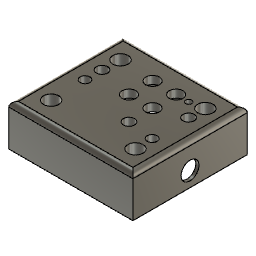
project (Autodesk Fusion 360 archive; units mm, degrees)
design "Obudowa"
Autodesk Fusion 360 part; units mm, degrees
sketch "Sketch1" plane through (0, 0, 0) normal (0, 0, 1) x (1, 0, 0)
  line L0 (-25, 25) -> (28.34, 25)
  line L1 (28.34, 25) -> (28.34, -20.72)
  line L2 (28.34, -20.72) -> (-25, -20.72)
  line L3 (-25, -20.72) -> (-25, 25)
  circle A0 centre (-19.67, -15.64) radius 1.6
  circle A1 centre (23.26, -15.64) radius 1.6
  circle A2 centre (23.26, 19.92) radius 1.6
  circle A3 centre (-19.793, 19.793) radius 1.6
  dimension "d1" = 53.34
  dimension "d2" = 45.72
  dimension "d3" = 3.2
  dimension "d4" = 5.08
  dimension "d5" = 5.33
  dimension "d6" = 3.2
  dimension "d7" = 3.2
  dimension "d8" = 3.2
  dimension "d9" = 5.08
  dimension "d10" = 5.08
  dimension "d11" = 5.207
  dimension "d12" = 5.207
  dimension "d13" = 5.08
  dimension "d14" = 5.08
  constraint horizontal L0
  constraint vertical L1
  constraint horizontal L2
  constraint vertical L3
  measures "d1" distance of L0.start L0.end
  measures "d2" distance of L0.start L2.end
  measures "d3" diameter of A0
  measures "d4" distance of L2 A0.centre
  measures "d5" distance of L3 A0.centre
  measures "d6" diameter of A1
  measures "d7" diameter of A2
  measures "d8" diameter of A3
  measures "d9" distance of L2 A1.centre
  measures "d10" distance of L0 A2.centre
  measures "d11" distance of L0 A3.centre
  measures "d12" distance of L3 A3.centre
  measures "d13" distance of L1 A2.centre
  measures "d14" distance of L1 A1.centre
extrude "Extrude1" add sketch "Sketch1" along normal blind 1.6 makes body 1
sketch "Sketch2" plane through (0, 0, 1.6) normal (0, 0, 1) x (-1, 0, 0)
  circle A0 centre (19.793, -19.793) radius 1.6
  circle A1 centre (-23.26, -19.92) radius 1.6
  circle A2 centre (-23.26, 15.64) radius 1.6
  circle A3 centre (19.67, 15.64) radius 1.6
  line L0 (25, 20.72) -> (-28.34, 20.72)
  line L1 (-28.34, 20.72) -> (-28.34, -25)
  line L2 (-28.34, -25) -> (25, -25)
  line L3 (25, -25) -> (25, 20.72)
  circle A4 centre (-3.94, -17.13) radius 2.2
  circle A5 centre (-11.8, 15.89) radius 4.25
  circle A6 centre (7.98, 9.3) radius 2.25
  dimension "d17" = 4.4
  dimension "d18" = 7.87
  dimension "d19" = 28.94
  dimension "d20" = 8.5
  dimension "d21" = 4.83
  dimension "d22" = 16.54
  dimension "d23" = 4.5
  dimension "d24" = 17.02
  dimension "d25" = 11.42
  measures "d17" diameter of A4
  measures "d18" distance of L2 A4.centre
  measures "d19" distance of L3 A4.centre
  measures "d20" diameter of A5
  measures "d21" distance of L0 A5.centre
  measures "d22" distance of L1 A5.centre
  measures "d23" diameter of A6
  measures "d24" distance of L3 A6.centre
  measures "d25" distance of L0 A6.centre
extrude "Extrude2" add sketch "Sketch2" along normal blind 12 contours A5 bodies 1
extrude "Extrude3" add sketch "Sketch2" along normal blind 8 contours A4 bodies 1
extrude "Extrude4" add sketch "Sketch2" along normal blind 8 contours A6 bodies 1
sketch "Sketch3" plane through (0, 0, 1.6) normal (0, 0, 1) x (-1, 0, 0)
  circle A0 centre (-18.865, -2.105) radius 1.65
  line L0 (-28.34, -25) -> (25, -25)
  line L1 (-28.34, 20.72) -> (-28.34, -25)
  circle A1 centre (-18.865, -2.105) radius 3.555
  line L2 (-18.865, -2.105) -> (-27.075, -2.105)
  line L3 (-27.075, -2.105) -> (-27.075, 1.45)
  line L4 (-27.075, 1.45) -> (-18.865, 1.45)
  line L5 (-18.865, 1.45) -> (-18.865, -2.105)
  line L6 (-18.865, -2.105) -> (-27.075, -2.105)
  line L7 (-27.075, -2.105) -> (-27.075, -5.66)
  line L8 (-27.075, -5.66) -> (-18.865, -5.66)
  line L9 (-18.865, -5.66) -> (-18.865, -2.105)
  dimension "d32" = 3.3
  dimension "d33" = 22.895
  dimension "d34" = 9.475
  dimension "d35" = 7.11
  dimension "d36" = 8.21
  dimension "d37" = 3.555
  dimension "d38" = 8.21
  dimension "d39" = 3.555
  constraint concentric A0 A1
  constraint horizontal L2
  constraint vertical L3
  constraint horizontal L4
  constraint vertical L5
  constraint coincident A0.centre A1.centre
  constraint horizontal L6
  constraint vertical L7
  constraint horizontal L8
  constraint vertical L9
  measures "d32" diameter of A0
  measures "d33" distance of A0.centre L0
  measures "d34" distance of A0.centre L1
  measures "d35" diameter of A1
  measures "d36" distance of A0.centre L2.end
  measures "d37" distance of A0.centre L4.end
  measures "d38" distance of A0.centre L2.end
  measures "d39" distance of A0.centre L8.end
extrude "Extrude5" add sketch "Sketch3" along normal blind 4.7 contours A0 A1 L5 L9 | A0 A1 L2 L5 L6 | A0 A1 L2 L6 L9 | A1 L2 L3 L4 L6 | A1 L2 L6 L7 L8 bodies 1
sketch "Sketch4" plane through (0, 0, 6.3) normal (0, 0, 1) x (-1, 0, 0)
  circle A0 centre (-18.865, -2.105) radius 1.65
  line L0 (-27.075, 1.45) -> (-27.075, -5.66)
  line L1 (-27.075, -5.66) -> (-18.865, -5.66)
  arc A1 (-18.865, -5.66) -> (-18.865, 1.45) centre (-18.865, -2.105) ccw
  line L2 (-18.865, 1.45) -> (-27.075, 1.45)
  line L3 (-25.3616, 1.45) -> (-28.1165, 1.45)
  line L4 (-28.1165, 1.45) -> (-28.1165, -5.66)
  line L5 (-28.1165, -5.66) -> (-25.3616, -5.66)
  line L6 (-25.3616, -5.66) -> (-25.3616, 1.45)
  dimension "d42" = 7.11
  constraint horizontal L3
  constraint vertical L4
  constraint horizontal L5
  constraint vertical L6
  constraint coincident L2 L3.start
  measures "d42" distance of L3.start L5.end
extrude "Extrude6" add sketch "Sketch4" along normal blind 5.71 contours L0 L1 L2 L3 L5 L6 | L0 L3 L4 L5 bodies 1
sketch "Sketch5" plane through (28.1165, 0, 0) normal (1, 0, 0) x (0, 1, 0)
  line L0 (-1.45, 6.3) -> (5.66, 6.3)
  line L1 (5.66, 6.3) -> (5.66, 12.01)
  line L2 (5.66, 12.01) -> (-1.45, 12.01)
  line L3 (-1.45, 12.01) -> (-1.45, 6.3)
  circle A0 centre (2.105, 8.58) radius 4.57
  line L4 (-20.72, 1.6) -> (25, 1.6)
  dimension "d45" = 9.14
  dimension "d46" = 3.555
  dimension "d47" = 6.98
  measures "d45" diameter of A0
  measures "d46" distance of L1 A0.centre
  measures "d47" distance of A0.centre L4
extrude "Extrude7" add sketch "Sketch5" along normal blind 15 contours L0 L1 L2 L3 A0 | L0 L1 L3 A0 | L2 A0 bodies 1
extrude "Extrude8" cut 1 faces at (26.2799, 3.1116, 12.01) along direction (0, 0, -1) blind 1.5 on bodies 1 bodies 1
sketch "FRONT" plane through (0, 0, 0) normal (0, 0, 1) x (1, 0, 0)
  line L0 (-28.33, 29.64) -> (31.67, 29.64)
  line L1 (31.67, 29.64) -> (31.67, -25.36)
  line L2 (31.67, -25.36) -> (-28.33, -25.36)
  line L3 (-28.33, -25.36) -> (-28.33, 29.64)
  line L4 (28.34, 25) -> (-25, 25)
  line L5 (28.34, -20.72) -> (28.34, 25)
  circle A0 centre (-2.33, 18.64) radius 3.45
  circle A1 centre (9.67, 18.64) radius 3.45
  circle A2 centre (-2.33, 6.64) radius 3.45
  circle A3 centre (9.67, 6.64) radius 3.45
  circle A4 centre (9.67, -5.36) radius 2.85
  circle A5 centre (22.9915, 11.64) radius 2.85
  circle A6 centre (16.0978, 18.6108) radius 1.55
  circle A7 centre (22.9591, -6.8283) radius 2.5
  circle A8 centre (-20.0454, 10.64) radius 2.85
  circle A9 centre (-20.0454, 1.9723) radius 2.5
  line L6 (-16, 15) -> (-16, 13) construction
  line L7 (-16, 13) -> (-14, 13) construction
  line L8 (-14, 13) -> (-14, 15) construction
  line L9 (-14, 15) -> (-16, 15) construction
  line L10 (26, -8) -> (26, -10) construction
  line L11 (26, -10) -> (27, -10) construction
  line L12 (27, -10) -> (27, -8) construction
  line L13 (27, -8) -> (26, -8) construction
  line L14 (26, 15) -> (26, 14) construction
  line L15 (26, 14) -> (27, 14) construction
  line L16 (27, 14) -> (27, 15) construction
  line L17 (27, 15) -> (26, 15) construction
  line L18 (9, 2) -> (9, 0) construction
  line L19 (9, 0) -> (10, 0) construction
  line L20 (10, 0) -> (10, 2) construction
  line L21 (10, 2) -> (9, 2) construction
  circle A10 centre (-19.67, -15.64) radius 1.6
  circle A11 centre (23.26, -15.64) radius 1.6
  circle A12 centre (23.26, 19.92) radius 1.6
  circle A13 centre (-19.79, 19.79) radius 1.6
  circle A14 centre (-19.79, 19.79) radius 3.85
  circle A15 centre (-19.79, 19.79) radius 5
  circle A16 centre (23.26, 19.92) radius 3.85
  circle A17 centre (23.26, 19.92) radius 5
  circle A18 centre (23.26, -15.64) radius 3.85
  circle A19 centre (23.26, -15.64) radius 5
  circle A20 centre (-19.67, -15.64) radius 3.85
  circle A21 centre (-19.67, -15.64) radius 5
  line L22 (-28.33, -25.36) -> (-29.93, -25.36)
  line L23 (-29.93, -25.36) -> (-29.93, 29.64)
  line L24 (-29.93, 29.64) -> (-28.33, 29.64)
  line L25 (-28.33, 29.64) -> (-28.33, -25.36)
  line L26 (-29.93, 29.64) -> (31.67, 29.64)
  line L27 (31.67, 29.64) -> (31.67, 31.24)
  line L28 (31.67, 31.24) -> (-29.93, 31.24)
  line L29 (-29.93, 31.24) -> (-29.93, 29.64)
  line L30 (31.67, 31.24) -> (33.27, 31.24)
  line L31 (33.27, 31.24) -> (33.27, -25.36)
  line L32 (33.27, -25.36) -> (31.67, -25.36)
  line L33 (31.67, -25.36) -> (31.67, 31.24)
  line L34 (-29.93, -25.36) -> (33.27, -25.36)
  line L35 (33.27, -25.36) -> (33.27, -26.96)
  line L36 (33.27, -26.96) -> (-29.93, -26.96)
  line L37 (-29.93, -26.96) -> (-29.93, -25.36)
  dimension "d52" = 60
  dimension "d53" = 55
  dimension "d54" = 4.64
  dimension "d55" = 3.33
  dimension "d56" = 6.9
  dimension "d59" = 6.9
  dimension "d60" = 12
  dimension "d62" = 6.9
  dimension "d63" = 6.9
  dimension "d64" = 12
  dimension "d65" = 5.7
  dimension "d66" = 12
  dimension "d67" = 5.7
  dimension "d68" = 3.1
  dimension "d69" = 5
  dimension "d70" = 5.7
  dimension "d71" = 5
  dimension "d72" = 3.2
  dimension "d73" = 3.2
  dimension "d74" = 3.2
  dimension "d75" = 3.2
  dimension "d76" = 7.7
  dimension "d77" = 10
  dimension "d78" = 7.7
  dimension "d79" = 10
  dimension "d80" = 7.7
  dimension "d81" = 10
  dimension "d82" = 7.7
  dimension "d83" = 10
  dimension "d92" = 1.6
  dimension "d93" = 55
  dimension "d94" = 61.6
  dimension "d95" = 1.6
  dimension "d96" = 1.6
  dimension "d97" = 56.6
  dimension "d98" = 63.2
  dimension "d99" = 1.6
  constraint horizontal L0
  constraint vertical L1
  constraint horizontal L2
  constraint vertical L3
  constraint concentric A13 A14
  constraint concentric A13 A15
  constraint concentric A12 A16
  constraint concentric A12 A17
  constraint concentric A11 A18
  constraint concentric A18 A19
  constraint concentric A10 A20
  constraint concentric A10 A21
  constraint horizontal L22
  constraint vertical L23
  constraint horizontal L24
  constraint vertical L25
  constraint horizontal L26
  constraint vertical L27
  constraint horizontal L28
  constraint vertical L29
  constraint horizontal L30
  constraint vertical L31
  constraint horizontal L32
  constraint vertical L33
  constraint horizontal L34
  constraint vertical L35
  constraint horizontal L36
  constraint vertical L37
  measures "d52" distance of L0.start L0.end
  measures "d53" distance of L0.start L2.end
  measures "d54" distance of L0 L4
  measures "d55" distance of L1 L5
  measures "d56" diameter of A0
  measures "d59" diameter of A1
  measures "d60" horizontal distance of A0.centre A1.centre
  measures "d62" diameter of A2
  measures "d63" diameter of A3
  measures "d64" horizontal distance of A3.centre A2.centre
  measures "d65" diameter of A4
  measures "d66" distance of A3.centre A4.centre
  measures "d67" diameter of A5
  measures "d68" diameter of A6
  measures "d69" diameter of A7
  measures "d70" diameter of A8
  measures "d71" diameter of A9
  measures "d72" diameter of A10
  measures "d73" diameter of A11
  measures "d74" diameter of A12
  measures "d75" diameter of A13
  measures "d76" diameter of A14
  measures "d77" diameter of A15
  measures "d78" diameter of A16
  measures "d79" diameter of A17
  measures "d80" diameter of A18
  measures "d81" diameter of A19
  measures "d82" diameter of A20
  measures "d83" diameter of A21
  measures "d92" distance of L2.end L22.end
  measures "d93" distance of L2.end L0.start
  measures "d94" distance of L23.end L0.end
  measures "d95" distance of L23.end L28.end
  measures "d96" distance of L27.end L30.end
  measures "d97" distance of L27.end L1.end
  measures "d98" distance of L22.end L31.end
  measures "d99" distance of L22.end L36.end
move_body "Move1" bodies 1 to x (1, 0, 0) y (0, 1, 0) z (0, 0, 1) at (0, 0, -18)
extrude "Extrude9" add sketch "FRONT" along normal blind 4 separate body contours L0 L1 L2 L3 L25 L26 L33 L34 | A15 | A17 | A19 | A21 makes body 2
move_body "Move2" bodies 1 to x (1, 0, 0) y (0, 1, 0) z (0, 0, 1) at (0, 0, -20)
extrude "Extrude10" add sketch "FRONT" against normal blind 16.4 contours A10 | A11 | A12 | A13 | A14 | A15 | A16 | A17 | A18 | A19 | A20 | A21 bodies 2
extrude "Extrude11" cut sketch "FRONT" against normal blind 34 contours A10 | A11 | A12 | A13 bodies 2
extrude "Extrude12" cut sketch "FRONT" against normal blind 15.8 contours A14 | A16 | A18 | A20 bodies 2
move_body "Move3" bodies 1 to x (1, 0, 0) y (0, 1, 0) z (0, 0, 1) at (0, 0, 20)
extrude "Extrude13" add sketch "FRONT" along normal blind 4 contours L0 L24 L26 L27 L28 L29 L33 | L3 L22 L23 L24 L25 L26 L34 | L1 L27 L30 L31 L32 L33 L34 | L2 L22 L32 L34 L35 L36 L37 bodies 2
extrude "Extrude14" add sketch "FRONT" against normal blind 17 separate body contours L0 L24 L26 L27 L28 L29 L33 | L3 L22 L23 L24 L25 L26 L34 | L1 L27 L30 L31 L32 L33 L34 | L2 L22 L32 L34 L35 L36 L37 makes body 3
combine "Combine1" operation add target body 3 tool bodies 2
sketch "Sketch7" plane through (0, 0, 0) normal (0, 0, -1) x (1, 0, 0)
  circle A0 centre (-2.33, -18.64) radius 3.45
  circle A1 centre (9.67, -18.64) radius 3.45
  circle A2 centre (-2.33, -6.64) radius 3.45
  circle A3 centre (9.67, -6.64) radius 3.45
  circle A4 centre (9.67, 5.36) radius 2.85
  circle A5 centre (22.9915, -11.64) radius 2.85
  circle A6 centre (16.0978, -18.6108) radius 1.55
  circle A7 centre (22.9591, 6.8283) radius 2.5
  circle A8 centre (-20.0454, -10.64) radius 2.85
  circle A9 centre (-20.0454, -1.9723) radius 2.5
  circle A10 centre (-19.79, -19.79) radius 5
  circle A11 centre (23.26, -19.92) radius 5
  circle A12 centre (-19.67, 15.64) radius 5
  circle A13 centre (23.26, 15.64) radius 5
  line L0 (-28.33, -29.64) -> (31.67, -29.64)
  line L1 (31.67, -29.64) -> (31.67, 25.36)
  line L2 (31.67, 25.36) -> (-28.33, 25.36)
  line L3 (-28.33, 25.36) -> (-28.33, -29.64)
  line L4 (23.26, -19.92) -> (22.46, -19.92)
  line L5 (22.46, -19.92) -> (22.46, -29.991)
  line L6 (22.46, -29.991) -> (23.26, -29.991)
  line L7 (23.26, -29.991) -> (23.26, -19.92)
  line L8 (23.26, -19.92) -> (24.06, -19.92)
  line L9 (24.06, -19.92) -> (24.06, -29.991)
  line L10 (24.06, -29.991) -> (23.26, -29.991)
  line L11 (23.26, -29.991) -> (23.26, -19.92)
  line L12 (23.26, -19.92) -> (32.3548, -19.92)
  line L13 (32.3548, -19.92) -> (32.3548, -20.72)
  line L14 (32.3548, -20.72) -> (23.26, -20.72)
  line L15 (23.26, -20.72) -> (23.26, -19.92)
  line L16 (23.26, -19.92) -> (32.3548, -19.92)
  line L17 (32.3548, -19.92) -> (32.3548, -19.12)
  line L18 (32.3548, -19.12) -> (23.26, -19.12)
  line L19 (23.26, -19.12) -> (23.26, -19.92)
  line L20 (32.3548, -19.92) -> (32.3548, -19.12)
  line L21 (23.26, 15.64) -> (22.46, 15.64)
  line L22 (22.46, 15.64) -> (22.46, 26.0742)
  line L23 (22.46, 26.0742) -> (23.26, 26.0742)
  line L24 (23.26, 26.0742) -> (23.26, 15.64)
  line L25 (24.06, 26.0742) -> (24.06, 15.64)
  line L26 (24.06, 15.64) -> (23.26, 15.64)
  line L27 (23.26, 15.64) -> (23.26, 26.0742)
  line L28 (23.26, 26.0742) -> (24.06, 26.0742)
  line L29 (23.26, 15.64) -> (32.1877, 15.64)
  line L30 (32.1877, 15.64) -> (32.1877, 14.84)
  line L31 (32.1877, 14.84) -> (23.26, 14.84)
  line L32 (23.26, 14.84) -> (23.26, 15.64)
  line L33 (23.26, 15.64) -> (32.1877, 15.64)
  line L34 (32.1877, 15.64) -> (32.1877, 16.44)
  line L35 (32.1877, 16.44) -> (23.26, 16.44)
  line L36 (23.26, 16.44) -> (23.26, 15.64)
  line L37 (-19.67, 15.64) -> (-30.1363, 15.64)
  line L38 (-30.1363, 15.64) -> (-30.1363, 14.84)
  line L39 (-30.1363, 14.84) -> (-19.67, 14.84)
  line L40 (-19.67, 14.84) -> (-19.67, 15.64)
  line L41 (-19.67, 15.64) -> (-30.1363, 15.64)
  line L42 (-30.1363, 15.64) -> (-30.1363, 16.44)
  line L43 (-30.1363, 16.44) -> (-19.67, 16.44)
  line L44 (-19.67, 16.44) -> (-19.67, 15.64)
  line L45 (-19.67, 15.64) -> (-18.87, 15.64)
  line L46 (-18.87, 15.64) -> (-18.87, 25.7874)
  line L47 (-18.87, 25.7874) -> (-19.67, 25.7874)
  line L48 (-19.67, 25.7874) -> (-19.67, 15.64)
  line L49 (-19.67, 15.64) -> (-20.47, 15.64)
  line L50 (-20.47, 15.64) -> (-20.47, 25.7874)
  line L51 (-20.47, 25.7874) -> (-19.67, 25.7874)
  line L52 (-19.67, 25.7874) -> (-19.67, 15.64)
  line L53 (-19.79, -19.79) -> (-20.59, -19.79)
  line L54 (-20.59, -19.79) -> (-20.59, -30.5224)
  line L55 (-20.59, -30.5224) -> (-19.79, -30.5224)
  line L56 (-19.79, -30.5224) -> (-19.79, -19.79)
  line L57 (-19.79, -19.79) -> (-18.99, -19.79)
  line L58 (-18.99, -19.79) -> (-18.99, -30.5512)
  line L59 (-18.99, -30.5512) -> (-19.79, -30.5512)
  line L60 (-19.79, -30.5512) -> (-19.79, -19.79)
  line L61 (-19.79, -19.79) -> (-29.2063, -19.79)
  line L62 (-29.2063, -19.79) -> (-29.2063, -20.59)
  line L63 (-29.2063, -20.59) -> (-19.79, -20.59)
  line L64 (-19.79, -20.59) -> (-19.79, -19.79)
  line L65 (-19.79, -19.79) -> (-29.2063, -19.79)
  line L66 (-29.2063, -19.79) -> (-29.2063, -18.99)
  line L67 (-29.2063, -18.99) -> (-19.79, -18.99)
  line L68 (-19.79, -18.99) -> (-19.79, -19.79)
  dimension "d104" = 0.8
  dimension "d105" = 0.8
  dimension "d106" = 0.8
  dimension "d107" = 0.8
  dimension "d108" = 0.8
  dimension "d109" = 0.8
  dimension "d110" = 0.8
  dimension "d111" = 0.8
  dimension "d112" = 0.8
  dimension "d113" = 0.8
  dimension "d114" = 0.8
  dimension "d115" = 0.8
  dimension "d116" = 0.8
  dimension "d117" = 0.8
  dimension "d118" = 0.8
  constraint horizontal L4
  constraint vertical L5
  constraint horizontal L6
  constraint vertical L7
  constraint coincident A11.centre L4.start
  constraint horizontal L8
  constraint vertical L9
  constraint horizontal L10
  constraint vertical L11
  constraint horizontal L12
  constraint vertical L13
  constraint horizontal L14
  constraint vertical L15
  constraint horizontal L16
  constraint vertical L17
  constraint horizontal L18
  constraint vertical L19
  constraint vertical L20
  constraint horizontal L21
  constraint vertical L22
  constraint horizontal L23
  constraint vertical L24
  constraint coincident A13.centre L21.start
  constraint horizontal L26
  constraint vertical L27
  constraint horizontal L28
  constraint vertical L25
  constraint horizontal L29
  constraint vertical L30
  constraint horizontal L31
  constraint vertical L32
  constraint horizontal L33
  constraint vertical L34
  constraint horizontal L35
  constraint vertical L36
  constraint horizontal L37
  constraint vertical L38
  constraint horizontal L39
  constraint vertical L40
  constraint coincident A12.centre L37.start
  constraint horizontal L41
  constraint vertical L42
  constraint horizontal L43
  constraint vertical L44
  constraint horizontal L45
  constraint vertical L46
  constraint horizontal L47
  constraint vertical L48
  constraint horizontal L49
  constraint vertical L50
  constraint horizontal L51
  constraint vertical L52
  constraint horizontal L53
  constraint vertical L54
  constraint horizontal L55
  constraint vertical L56
  constraint coincident A10.centre L53.start
  constraint horizontal L57
  constraint vertical L58
  constraint horizontal L59
  constraint vertical L60
  constraint horizontal L61
  constraint vertical L62
  constraint horizontal L63
  constraint vertical L64
  constraint horizontal L65
  constraint vertical L66
  constraint horizontal L67
  constraint vertical L68
  measures "d104" distance of A11.centre L4.end
  measures "d105" distance of A11.centre L8.end
  measures "d106" distance of A11.centre L14.end
  measures "d107" distance of A11.centre L18.end
  measures "d108" distance of A13.centre L21.end
  measures "d109" distance of A13.centre L25.end
  measures "d110" distance of A13.centre L31.end
  measures "d111" distance of A13.centre L35.end
  measures "d112" distance of A12.centre L39.end
  measures "d113" distance of A12.centre L43.end
  measures "d114" distance of A12.centre L45.end
  measures "d115" distance of A12.centre L49.end
  measures "d116" distance of A10.centre L53.end
  measures "d117" distance of A10.centre L63.end
  measures "d118" distance of A10.centre L67.end
extrude "Extrude15" add sketch "Sketch7" along normal blind 15 contours A10 L3 L61 L65 L67 | A10 L0 L56 L58 L60 | A10 L3 L61 L63 L65 | A10 L0 L54 L56 L60 | A12 L3 L37 L39 L41 | A11 L0 L5 L7 L11 | A12 L3 L37 L41 L43 | A11 L0 L7 L9 L11 | A11 L1 L12 L16 L18 | A12 L2 L46 L48 L52 | A11 L1 L12 L14 L16 | A12 L2 L48 L50 L52 | A13 L1 L29 L31 L33 | A13 L2 L22 L24 L27 | A13 L1 L29 L33 L35 | A13 L2 L24 L25 L27 bodies 3
fillet "Fillet1" radius 2.5 4 edges at (1.67, -26.96, 4) (-29.93, 2.14, 4) (1.67, 31.24, 4) (33.27, 2.14, 4) on bodies 3
move_body "Move4" bodies 1 3 to x (1, 0, 0) y (0, 1, 0) z (0, 0, 1) at (0, 0, 18)
sketch "Sketch8" plane through (0, 0, 0) normal (0, 0, 1) x (1, 0, 0)
  line L0 (-29.93, -26.96) -> (33.27, -26.96)
  line L1 (33.27, -26.96) -> (33.27, 31.24)
  line L2 (33.27, 31.24) -> (-29.93, 31.24)
  line L3 (-29.93, 31.24) -> (-29.93, -26.96)
  line L4 (31.67, 29.64) -> (-28.33, 29.64)
  line L5 (-28.33, 29.64) -> (-28.33, -25.36)
  line L6 (-28.33, -25.36) -> (31.67, -25.36)
  line L7 (31.67, -25.36) -> (31.67, 29.64)
  circle A0 centre (-19.67, -15.65) radius 1.6
  circle A1 centre (23.26, -15.64) radius 1.6
  circle A2 centre (23.26, 19.92) radius 1.6
  circle A3 centre (-19.79, 19.79) radius 1.6
  circle A4 centre (-19.67, -15.65) radius 3.55
  circle A5 centre (23.26, -15.64) radius 3.55
  circle A6 centre (23.26, 19.92) radius 3.55
  circle A7 centre (-19.79, 19.79) radius 3.55
  dimension "d123" = 3.2
  dimension "d124" = 3.2
  dimension "d125" = 3.2
  dimension "d126" = 7.1
  dimension "d127" = 7.1
  dimension "d128" = 7.1
  dimension "d129" = 7.1
  constraint horizontal L0
  constraint vertical L1
  constraint horizontal L2
  constraint vertical L3
  constraint horizontal L4
  constraint vertical L5
  constraint horizontal L6
  constraint vertical L7
  constraint concentric A0 A4
  constraint concentric A1 A5
  constraint concentric A2 A6
  constraint concentric A3 A7
  measures "d123" diameter of A0
  measures "d124" diameter of A2
  measures "d125" diameter of A3
  measures "d126" diameter of A4
  measures "d127" diameter of A5
  measures "d128" diameter of A6
  measures "d129" diameter of A7
move_body "Move5" bodies 1 3 to x (1, 0, 0) y (0, 1, 0) z (0, 0, 1) at (0, 0, 5.1)
extrude "Extrude16" add sketch "Sketch8" along normal blind 1.6 separate body contours L0 L1 L2 L3 | L4 L5 L6 L7 | A4 | A5 | A6 | A7 makes body 4
move_body "Move6" bodies 1 to x (1, 0, 0) y (0, 1, 0) z (0, 0, 1) at (0, 0, 1)
extrude "Extrude17" add sketch "Sketch8" along normal blind 5.1 contours A4 | A5 | A6 | A7 bodies 4
move_body "Move7" bodies 1 to x (1, 0, 0) y (0, 1, 0) z (0, 0, 1) at (0, 0, -1)
extrude "Extrude18" add sketch "Sketch8" along normal blind 6.1 contours L0 L1 L2 L3 bodies 4
fillet "Fillet2" radius 2.5 4 edges at (33.27, 2.14, 0) (1.67, -26.96, 0) (-29.93, 2.14, 0) (1.67, 31.24, 0) on bodies 4
combine "Combine2" operation cut target body 3 tool bodies 1 keep tools
hidden bodies 1 4
named bodies: "PCB"
